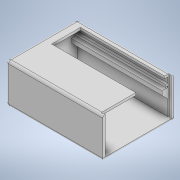
# Autodesk Inventor part: Case
Saved by Autodesk Inventor 2020 (Build 240168000, 168)
## iProperties
Created: 2019-09-29
Part Number: Case
Material: Generic
Document SubType Name: Modeling
Designer: bzs3334
Density: 1 g/cm^3
Appearance: Default
Author: bzs3334
Autodesk Inventor part; units mm, degrees
ref_plane "YZ Plane" through (0, 0, 0) normal (1, 0, 0) x (0, 1, 0)
ref_plane "XZ Plane" through (0, 0, 0) normal (0, 1, 0) x (-1, 0, 0)
ref_plane "XY Plane" through (0, 0, 0) normal (0, 0, 1) x (1, 0, 0)
sketch "Sketch1" plane through (0, 0, 0) normal (0, 1, 0) x (-1, 0, 0)
  line L0 (55, -40) -> (-55, -40)
  line L1 (-55, -40) -> (-55, 40)
  line L2 (-55, 40) -> (55, 40)
  line L3 (55, 40) -> (55, -40)
  line L4 (-58, -43) -> (58, -43)
  line L5 (58, -43) -> (58, 43)
  line L6 (58, 43) -> (-58, 43)
  line L7 (-58, 43) -> (-58, -43)
  point P0 (0, 0)
  dimension "d0" = 110
  dimension "d1" = 55
  dimension "d2" = 80
  dimension "d3" = 40
  dimension "d4" = 3
  constraints: 16 end point, 4 parallel, 2 perpendicular, 1 horizontal, 3 other
  measures "d0" distance of L0.start L0.end
  measures "d1" horizontal distance of L0.start point (0, 0)
  measures "d2" distance of L2.end L0.start
  measures "d3" vertical distance of L0.start point (0, 0)
  measures "d4" distance between parallel lines of L4 L0
extrude "Extrusion1" add sketch "Sketch1" against normal blind 3 contours L0 L1 L2 L3 | L7 L6 L5 L4
extrude "Extrusion2" add sketch "Sketch1" along normal blind 45
sketch "Sketch4" plane through (58, -3, 43) normal (1, 0, 0) x (0, 0, -1)
  line L0 (0, 0) -> (0, 48) projected
  line L1 (86, 0) -> (0, 0) projected
  line L2 (86, 0) -> (86, 48) projected
  line L3 (0, 48) -> (86, 48) projected
  point P0 (43, 3)
extrude "Extrusion3" cut sketch "Sketch4" against normal blind 3
sketch "Sketch5" plane through (0, 45, 0) normal (0, 1, 0) x (1, 0, 0)
  line L0 (55, 43) -> (-58, 43) projected
  line L1 (-58, 43) -> (-58, -43) projected
  line L2 (-58, -43) -> (55, -43) projected
  line L3 (55, 43) -> (55, -43) projected
  line L4 (55, 36) -> (-47, 36)
  line L5 (-47, 36) -> (-47, 1)
  line L6 (-47, 1) -> (55, 1)
  line L7 (55, 1) -> (55, 36)
  line L8 (-55, 40) -> (55, 40) projected
  line L9 (-55, -40) -> (-55, 40) projected
  point P0 (0, 0)
  point P1 (55, 1)
  dimension "d11" = 4
  dimension "d12" = 8
  dimension "d13" = 35
  constraints: 8 end point, 2 parallel, 1 horizontal, 1 perpendicular, 1 point on line
  measures "d11" distance between parallel lines of L8 L4
  measures "d12" distance between parallel lines of L9 L5
  measures "d13" distance of L4.end L5.end
extrude "Extrusion4" add sketch "Sketch5" against normal blind 3 contours L3 L4 L5 L6 L2 L1 L0
sketch "Sketch6" plane through (55, -3, 43) normal (1, 0, 0) x (0, 0, -1)
  line L0 (0, 48) -> (44, 48) projected
  line L1 (86, 48) -> (86, 0) projected
  line L2 (0, 48) -> (86, 48)
  line L3 (86, 48) -> (86, 0)
  line L4 (86, 0) -> (0, 0)
  line L5 (0, 0) -> (0, 48)
  line L6 (0, 0) -> (0, 48) projected
  line L7 (86, 0) -> (0, 0) projected
  line L8 (86, 48) -> (86, 0) projected
  line L9 (79, 48) -> (86, 48) projected
  line L10 (79, 48) -> (79, 45) projected
  line L11 (83, 45) -> (79, 45) projected
  line L12 (83, 3) -> (83, 45) projected
  line L13 (3, 3) -> (83, 3) projected
  line L14 (3, 3) -> (3, 45) projected
  line L15 (44, 45) -> (3, 45) projected
  line L16 (44, 48) -> (44, 45) projected
  line L17 (0, 48) -> (44, 48) projected
  line L18 (44, 48) -> (44, 45) projected
  line L19 (44, 48) -> (79, 48)
  line L20 (79, 48) -> (79, 45)
  line L21 (79, 45) -> (44, 45)
  line L22 (44, 45) -> (44, 48)
  line L23 (44, 45) -> (3, 45) projected
  line L24 (3, 45) -> (3, 48)
  line L25 (83, 45) -> (79, 45) projected
  line L26 (83, 45) -> (83, 48)
  line L27 (79, 48) -> (86, 48) projected
  point P0 (43, 3)
  constraints: 20 end point, 4 parallel, 4 perpendicular, 2 horizontal, 2 point on line
extrude "Extrusion5" add sketch "Sketch6" along normal blind 4 contours L0 L24 L14 L13 L12 L26 L2 L1 L4 L5
sketch "Sketch7" plane through (0, 45, 0) normal (0, 1, 0) x (1, 0, 0)
  line L0 (55, -40) -> (59, -40) projected
  line L1 (55, -40) -> (57, -40)
  line L2 (57, -40) -> (57, -41)
  line L3 (57, -41) -> (55, -41)
  line L4 (55, -41) -> (55, -40)
  line L5 (84.8, 0) -> (-81.8, 0) projected
  line L6 (-81.8, 0) -> (84.8, 0) projected
  line L7 (55, 40) -> (57, 40)
  line L8 (57, 40) -> (57, 41)
  line L9 (57, 41) -> (55, 41)
  line L10 (55, 41) -> (55, 40)
  point P0 (0, 0)
  dimension "d18" = 2
  dimension "d19" = 1
  constraints: 16 end point, 4 symmetric about line, 2 parallel, 1 horizontal, 1 perpendicular
  measures "d18" distance of L2.end L3.end
  measures "d19" distance of L3.end L0.start
extrude "Extrusion6" cut sketch "Sketch7" against normal up to surface (45 mm away)
sketch "Sketch8" plane through (-58, -3, -43) normal (-1, 0, 0) x (0, 0, 1)
  line L0 (51.5, 18) -> (66.5, 18)
  line L1 (66.5, 18) -> (66.5, 3)
  line L2 (66.5, 3) -> (51.5, 3)
  line L3 (51.5, 3) -> (51.5, 18)
  line L4 (23, 18) -> (35, 18)
  line L5 (35, 18) -> (35, 3)
  line L6 (35, 3) -> (23, 3)
  line L7 (23, 3) -> (23, 18)
  line L8 (86, 48) -> (86, 0) projected
  line L9 (86, 0) -> (0, 0) projected
  line L10 (0, 0) -> (0, 48) projected
  point P0 (29, 18)
  point P1 (59, 18)
  point P2 (23, 10.5)
  point P3 (51.5, 10.5)
  dimension "d23" = 15
  dimension "d25" = 15
  dimension "d26" = 12
  dimension "d28" = 27
  dimension "d29" = 29
  dimension "d31" = 3
  constraints: 16 end point, 4 midpoint, 4 parallel, 2 horizontal, 2 perpendicular, 1 collinear, 1 point on line
  measures "d23" distance of L0.start L0.end
  measures "d25" distance of L2.end L0.start
  measures "d26" distance of L4.start L4.end
  measures "d28" distance from line of L8 point (59, 18)
  measures "d29" distance from line of L10 point (29, 18)
  measures "d31" distance between parallel lines of L9 L2
extrude "Extrusion7" cut sketch "Sketch8" against normal blind 4
fillet "Fillet2" radius 3 9 edges at (0.5, 45, 43) (0.5, -3, 43) (0.5, -3, -43) (-58, -3, 0) (-58, 21, 43) (-58, 45, 0) (0.5, 45, -43) (-58, 21, -43) (59, -3, 0)
sketch "Sketch9" plane through (0, 0, 0) normal (0, 1, 0) x (1, 0, 0)
  line L0 (-6, -6.25) -> (6, -6.25)
  line L1 (6, -6.25) -> (6, 5.75)
  line L2 (6, 5.75) -> (-6, 5.75)
  line L3 (-6, 5.75) -> (-6, -6.25)
  line L4 (-55, 8) -> (-55, -8.5) projected
  line L5 (-55, -0.25) -> (-6, -0.25)
  line L6 (-58, 8) -> (-55, 8) projected
  point P0 (0, 0)
  dimension "d36" = 12
  dimension "d37" = 12
  dimension "d38" = 6
  constraints: 10 end point, 3 parallel, 2 midpoint, 1 horizontal, 1 perpendicular
  measures "d36" distance of L2.end L0.start
  measures "d37" distance of L1.end L2.end
  measures "d38" distance from line of L1 point (0, 0)
extrude "Extrusion8" add sketch "Sketch9" along normal blind 7
sketch "Sketch11" plane through (-6, 0, -5.75) normal (-1, 0, 0) x (0, 0, 1)
  line L0 (12, 0) -> (0, 0) projected
  line L1 (12, 0) -> (12, 7) projected
  line L2 (0, 7) -> (12, 7) projected
  line L3 (0, 0) -> (0, 7) projected
  point P0 (5.75, 0)
extrude "Extrusion10" add sketch "Sketch11" along normal up to surface (52 mm away)
sketch "Sketch12" plane through (-55, 0, -40) normal (0, 0, 1) x (1, 0, 0)
  line L0 (114, 42) -> (0, 42) projected
  line L1 (114, 0) -> (114, 42) projected
  line L2 (0, 0) -> (114, 0) projected
  line L3 (0, 42) -> (0, 0) projected
  line L4 (0, 42) -> (0, 0) projected
  line L5 (110, 44.8284) -> (110, 0) projected
  line L6 (0, 31) -> (110, 31)
  line L7 (110, 31) -> (110, 26)
  line L8 (110, 26) -> (0, 26)
  line L9 (0, 26) -> (0, 31)
  point P0 (55, 0)
  point P1 (0, 26)
  dimension "d46" = 11
  dimension "d47" = 5
  constraints: 8 end point, 2 parallel, 2 point on line, 1 horizontal, 1 perpendicular
  measures "d46" distance between parallel lines of L0 L6
  measures "d47" distance between parallel lines of L8 L6
extrude "Extrusion11" add sketch "Sketch12" along normal blind 7 contours L5 L8 L3 L6
chamfer "Chamfer1" distance 7 angle 45 1 edges at (0, 26, -40)
mirror "Mirror1" about plane through (0, 0, 0) normal (0, 0, 1) of "Extrusion11"
sketch "Sketch13" plane through (55, -3, 43) normal (1, 0, 0) x (0, 0, -1)
  line L0 (10, 29) -> (10, 34) projected
  line L1 (3, 34) -> (10, 34) projected
  line L2 (3, 29) -> (10, 29) projected
  line L3 (10, 29) -> (3, 29) projected
  line L4 (3, 29) -> (3, 34)
  line L5 (3, 3) -> (3, 48) projected
  point P0 (43, 3)
  constraints: 2 end point, 1 collinear
extrude "Extrusion12" cut sketch "Sketch13" against normal blind 85
sketch "Sketch14" plane through (-55, 26, 33) normal (0, 0, -1) x (-1, 0, 0)
  point P0 (-55, -26)
sketch "Sketch15" plane through (-55, 26, 33) normal (0, 0, -1) x (-1, 0, 0)
  line L0 (0, 0) -> (-25, 0) projected
  line L1 (-25, 5) -> (0, 5) projected
  line L2 (-25, 0) -> (-25, 5) projected
  line L3 (0, -26) -> (0, 16) projected
  point P0 (-55, -26)
extrude "Extrusion13" add sketch "Sketch15" along normal blind 5
chamfer "Chamfer2" distance 7 angle 45 1 edges at (-42.5, 26, 40)
sketch "Sketch16" plane through (-55, 42, -40) normal (0, 0, 1) x (1, 0, 0)
  line L0 (0, -16) -> (0, -11) projected
  line L1 (0, -16) -> (110, -16) projected
  line L2 (110, -16) -> (110, -11) projected
  line L3 (110, -11) -> (0, -11) projected
  line L4 (110, 0) -> (8, 0) projected
  line L5 (0, -11) -> (0, 0) projected
  line L6 (110, -11) -> (110, 0) projected
  line L7 (110, 2.8284) -> (110, -42) projected
  line L8 (0, -6.5) -> (110, -6.5)
  line L9 (110, -6.5) -> (110, -9.5)
  line L10 (110, -9.5) -> (0, -9.5)
  line L11 (0, -9.5) -> (0, -6.5)
  point P0 (55, -42)
  point P1 (0, -9.5)
  point P2 (110, -9.5)
  point P3 (110, -6.5)
  dimension "d60" = 1.5
  dimension "d61" = 3
  constraints: 8 end point, 2 parallel, 2 point on line, 1 horizontal, 1 perpendicular
  measures "d60" distance between parallel lines of L10 L3
  measures "d61" distance of L10.end L8.start
extrude "Extrusion14" add sketch "Sketch16" along normal blind 3 contours L5 L8 L6 L10
sketch "Sketch17" plane through (55, 0, 40) normal (0, 0, -1) x (-1, 0, 0)
  line L0 (85, 26) -> (110, 26) projected
  line L1 (110, 31) -> (110, 26) projected
  line L2 (110, 31) -> (85, 31) projected
  line L3 (85, 31) -> (85, 26) projected
  line L4 (0, 45) -> (102, 45) projected
  line L5 (0, 45) -> (0, 42) projected
  line L6 (102, 42) -> (0, 42) projected
  line L7 (102, 45) -> (102, 42) projected
  line L8 (110, 0) -> (110, 42) projected
  line L9 (110, 32.5) -> (94.2848, 32.5)
  line L10 (94.2848, 32.5) -> (94.2848, 35.5)
  line L11 (94.2848, 35.5) -> (110, 35.5)
  line L12 (110, 35.5) -> (110, 32.5)
  point P0 (55, 0)
  dimension "d64" = 1.5
  dimension "d65" = 3
  constraints: 8 end point, 2 parallel, 1 horizontal, 1 perpendicular, 1 point on line
  measures "d64" distance between parallel lines of L9 L2
  measures "d65" distance of L9.end L10.end
extrude "Extrusion15" add sketch "Sketch17" along normal blind 9 contours L9 L10 L11 L8
equation "\"d1\" = 0.5 * d0"
equation "\"d3\" = 0.5 * d2"
equation "\"d38\" = 0.5 * d37"
body "Solid1"
